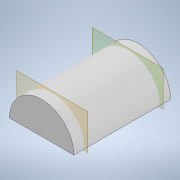
# Autodesk Inventor part: chestTop
Saved by Autodesk Inventor 2020.3 (Build 243373000, 373)
## iProperties
Created: 2021-02-24
Part Number: chestTop
Material: Generic
Document SubType Name: Modeling
Designer: con_c_000
Density: 1 g/cm^3
Appearance: Default
Author: con_c_000
Autodesk Inventor part; units mm, degrees
ref_plane "YZ Plane" through (0, 0, 0) normal (1, 0, 0) x (0, 1, 0)
ref_plane "XZ Plane" through (0, 0, 0) normal (0, 1, 0) x (-1, 0, 0)
ref_plane "XY Plane" through (0, 0, 0) normal (0, 0, 1) x (1, 0, 0)
sketch "Sketch1" plane through (0, 0, 0) normal (0, 0, 1) x (1, 0, 0)
  arc A0 (598.1223, 0) -> (-11.4777, 0) centre (293.3223, 0) ccw
  line L0 (-11.4777, 0) -> (598.1223, 0)
  point P0 (0, 0)
  dimension "d0" = 609.6
  dimension "d1" = 304.8
  constraints: 2 end point, 2 point on circle, 1 centre point, 1 horizontal
  measures "d0" distance of L0.start L0.end
  measures "d1" radius of A0
extrude "Extrusion1" add sketch "Sketch1" along normal blind 914.4
shell "Shell1" thickness 12.7 removed faces 1 at (191.7223, 0, 609.6)
ref_plane "Work Plane1" through (0, 0, 812.8) normal (0, 0, 1) x (1, 0, 0)
ref_plane "Work Plane2" through (0, 0, 101.6) normal (0, 0, -1) x (-1, 0, 0)
sketch "Sketch2" plane through (0, 0, 101.6) normal (0, 0, -1) x (-1, 0, 0)
  circle A0 centre (17.8277, 0) radius 10.16
  circle A1 centre (17.8277, 0) radius 6.35
  arc A2 (11.4777, 0) -> (-598.1223, 0) centre (-293.3223, 0) ccw projected
  point P0 (0, 0)
  dimension "d7" = 20.32
  dimension "d8" = 12.7
  constraints: 2 centre point, 1 coincident, 1 tangent
  measures "d7" diameter of A0
  measures "d8" diameter of A1
extrude "Extrusion2" add sketch "Sketch2" against normal blind 50.8
sketch "Sketch3" plane through (0, 0, 812.8) normal (0, 0, 1) x (1, 0, 0)
  arc A0 (-11.3766, 7.8491) -> (-7.6677, 0) centre (-17.8277, 0) ccw projected
  circle A1 centre (-17.8277, 0) radius 10.16
  circle A2 centre (-17.8277, 0) radius 6.35
  point P0 (0, 0)
  point P1 (-7.6677, 0)
  dimension "d11" = 12.7
  constraints: 2 centre point, 2 coincident, 1 concentric
  measures "d11" diameter of A2
extrude "Extrusion3" add sketch "Sketch3" against normal blind 50.8
body "Solid1"
